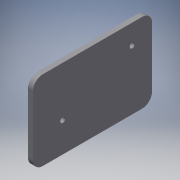
# Autodesk Inventor part: Base
Saved by Autodesk Inventor 2016 (Build 200138000, 138)
## iProperties
Created: 2014-03-13
Part Number: Base
Material: Generic
Document SubType Name: Modeling
Designer: John
Density: 1 g/cm^3
Appearance: Default
Author: John
Autodesk Inventor part; units mm, degrees
ref_plane "YZ Plane" through (0, 0, 0) normal (1, 0, 0) x (0, 1, 0)
ref_plane "XZ Plane" through (0, 0, 0) normal (0, 1, 0) x (-1, 0, 0)
ref_plane "XY Plane" through (0, 0, 0) normal (0, 0, 1) x (1, 0, 0)
sketch "Sketch1" plane through (0, 0, 0) normal (1, 0, 0) x (0, 1, 0)
  line L0 (0, 0) -> (50.8, 0)
  line L1 (50.8, 0) -> (50.8, 76.2)
  line L2 (50.8, 76.2) -> (0, 76.2)
  line L3 (0, 76.2) -> (0, 0)
  dimension "d0" = 50.8
  dimension "d1" = 76.2
  constraints: 8 end point, 2 parallel, 1 horizontal, 1 perpendicular
  measures "d0" distance of L2.end L1.end
  measures "d1" distance of L1.end L0.end
extrude "Extrusion1" add sketch "Sketch1" along normal blind 3.175
sketch "Sketch2" plane through (3.175, 0, 0) normal (1, 0, 0) x (0, 0, -1)
  line L0 (0, 0) -> (0, 50.8) projected
  line L1 (0, 50.8) -> (-76.2, 50.8) projected
  line L2 (-76.2, 50.8) -> (-76.2, 0) projected
  point P0 (-57.15, 19.05)
  point P1 (-12.7, 38.1)
  dimension "d4" = 12.7
  dimension "d5" = 12.7
  dimension "d6" = 31.75
  dimension "d7" = 19.05
  measures "d4" distance from line of L0 point (-12.7, 38.1)
  measures "d5" distance from line of point (-12.7, 38.1) L1
  measures "d6" distance from line of L1 point (-57.15, 19.05)
  measures "d7" distance from line of L2 point (-57.15, 19.05)
hole "Hole1" at (3.175, 19.05, 57.15) at (3.175, 38.1, 12.7) direction (-1, 0, 0) diameter 3.175 end through all
fillet "Fillet1" radius 6.35 4 edges at (1.5875, 50.8, 76.2) (1.5875, 0, 76.2) (1.5875, 0, 0) (1.5875, 50.8, 0)
body "Solid1"
